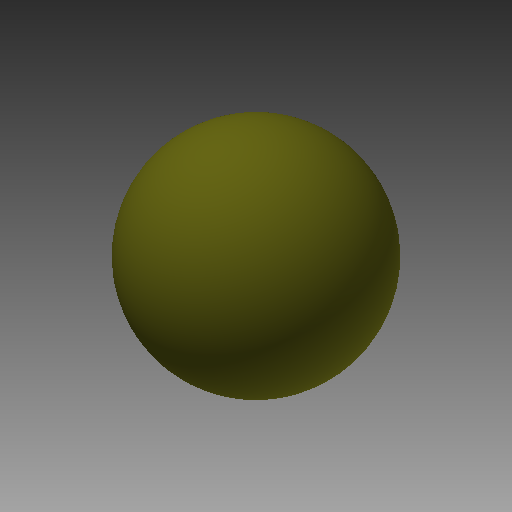
# Autodesk Inventor part: 6205_PART3
Saved by Autodesk Inventor 2018 (Build 220112000, 112)
## iProperties
Category: PARTsolutions
Company: SKF
Created: 2018-05-05
Part Number: 6205_PART3
Catalog Web Link: www.cadenas.de
Description: -Deep groove ball bearings, single row
Vendor: SKF
Document SubType Name: Modeling
Designer: psAdmin
Manufacturer: SKF
Mass: 0.261898 g
Surface Area: 1.97958 cm^2
Volume: 0.261898 cm^3
Density: 1 g/cm^3
Material: Generic
Appearance: PSOLRGB-191-191-0
PSOL_IDENT_0: {$CADENAS_DATA\23d-libs\skf\bearings_units_and_housings\ball_bearings\deep_groove_ball_bearings\deep
PSOL_IDENT_1: _groove_ball_bearings_single_row\bb1_001_101.prj},190 {VTYP=3D},{NB=6205_PART3},{LINA=6205_PART3},{N
PSOL_IDENT_2: N=BB1_001_101_PART3},{NOPRJ=TRUE},{DATE=14.07.2017 09:01:20},{GEOMDATE=14.07.2017 08:21:21},{VERSION=
PSOL_IDENT_3: },{LINEID=214770},{LINESUBID=-1},{WBVAR=}  {NB=6205_PART3},{LINA=6205_PART3},{KT=DUMMY},{PRODUCTID=1
PSOL_IDENT_4: 050010205},{DESIGNATION=6205},{DD=25.000},{D=52.000},{B=15.000},{HH=-1000000015047466219876688855040
PSOL_IDENT_5: .000},{DD1=34.350},{DD2=-1000000015047466219876688855040.000},{DD22=-1000000015047466219876688855040
PSOL_IDENT_6: .000},{D1=43.950},{D2=46.210},{BB=-1000000015047466219876688855040.000},{R12=1},{R121=1.000},{R122=1
PSOL_IDENT_7: .000},{LOAD1=14.800},{LOAD2=7.800},{LOAD3=0.335},{SPEED1=28000},{SPEED2=18000},{MASS=0.128},{PITCH=3
PSOL_IDENT_8: 9.040},{DW=7.938},{Z=9.000},{II=1.000},{TYPEID=105001},{HELP=4.025},{HELP2=2.895},{DD1ALG=17.175},{T
PSOL_IDENT_9: AXONOMY=1},{DESIGN=dgbb1},{MAPPING=BCZ50,DESIGNATION|IRD01,DD|ORD10,D|BCW30,B|ORL64,HH|IRD30,DD1|IRD
PSOL_IDENT_10: 46,DD2|IRD43,DD22|ORD30,D1|ORD43,D2|ORL60,BB|ORL03,R121|BCE41,R122|BCC02,LOAD1|BCC16,LOAD2|BCC12,LOA
PSOL_IDENT_11: D3|BCC43,SPEED1|BCC45,SPEED2|BCM01,MASS|BCD50,PITCH|RBD10,DW|BCN81,Z|BCN80,II},{DESIGNLIST=dgbbrs,dg
PSOL_IDENT_12: bb1,dgbb2rs,dgbb2z,dgbbn1,dgbbz},{YALG=17.17500},{HALG=4.67500},{YALG1=21.97500},{HALG1=4.02500},{PI
PSOL_IDENT_13: TCH1=39.04000},{DW1=7.93800},{SH=17.175},{CU=1.4124},{SORT=DD},{PIM=6205}
NT: Deep groove ball bearings, single row
NB: 6205_PART3
NBSYN: $DESIGNATION._PART3
LINA: 6205_PART3
DESIGNATION: 6205
DD: 25.000
D: 52.000
B: 15.000
LOAD1: 14.800
LOAD2: 7.800
LOAD3: 0.335
SPEED1: 28000
SPEED2: 18000
SUPPLIER: SKF
ARTICLENO: 6205_PART3
BOMINFO: 6205_PART3
CREATOR: CADENAS GmbH
Title: 6205_PART3
Author: Cadenas PARTsolutions
Comments: Deep groove ball bearings, single row
Autodesk Inventor part; units mm, degrees
ref_plane "YZ Plane" through (0, 0, 0) normal (1, 0, 0) x (0, 1, 0)
ref_plane "XZ Plane" through (0, 0, 0) normal (0, 1, 0) x (-1, 0, 0)
ref_plane "XY Plane" through (0, 0, 0) normal (0, 0, 1) x (1, 0, 0)
sketch "Sketch_1" plane through (0, 0, 0) normal (0, 0, 1) x (1, 0, 0)
  line L0 (11.469, 19.52) -> (3.531, 19.52)
  arc A0 (11.469, 19.52) -> (3.531, 19.52) centre (7.5, 19.52) ccw
  line L1 (11.469, 19.52) -> (3.531, 19.52)
  dimension "d0" = 360
  constraints: 4 end point, 2 point on circle, 1 centre point
revolve "Revolution1" add sketch "Sketch_1" angle 360 about axis through (11.469, 19.52, 0) along (1, 0, 0)
body "Solid1"
